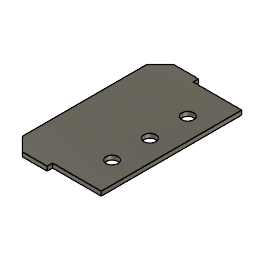
GPL H300 to 300G17_ (Autodesk Fusion 360 design; units mm, degrees)
Autodesk Fusion 360 part; units mm, degrees
sketch "スケッチ1" plane through (0, 0, 0) normal (0, 0, 1) x (1, 0, 0)
  line L0 (-9.5, 140) -> (-80.5, 140)
  line L1 (-80.5, 140) -> (-80.5, -140)
  line L2 (-80.5, -140) -> (-9.5, -140)
  line L3 (80.5, -130) -> (80.5, 130)
  line L4 (74.75, 130) -> (-80.5, -140) construction
  line L5 (-80.5, 140) -> (74.75, -130) construction
  line L6 (-9.5, 140) -> (-9.5, 130)
  line L7 (-9.5, 130) -> (80.5, 130)
  line L8 (-9.5, -140) -> (-9.5, -130)
  line L9 (-9.5, -130) -> (80.5, -130)
  dimension "d2" = 280
  constraint horizontal L0
  constraint perpendicular L0 L1
  constraint parallel L0 L2
  constraint parallel L1 L3
  constraint coincident L4 origin
  constraint coincident L5 origin
  constraint vertical L6
  constraint horizontal L7
  constraint vertical L8
  constraint horizontal L9
  constraint coincident L7 L4.start
  constraint coincident L9 L5.end
  measures "d2" distance of L0.end L1.end
extrude "押し出し1" add sketch "スケッチ1" along normal blind 8
chamfer "面取り1" distance 25 angle 45 2 edges at (-80.5, -140, 4) (-80.5, 140, 4)
sketch "スケッチ2" plane through (0, 0, 8) normal (0, 0, 1) x (-1, 0, 0)
  line L0 (55.5, -140) -> (80.5, -115)
  line L1 (80.5, -115) -> (80.5, 115)
  line L2 (80.5, 115) -> (55.5, 140)
  line L3 (55.5, 140) -> (9.5, 140)
  line L4 (9.5, 140) -> (9.5, 130)
  line L5 (9.5, 130) -> (-80.5, 130)
  line L6 (-80.5, 130) -> (-80.5, -130)
  line L7 (-80.5, -130) -> (9.5, -130)
  line L8 (9.5, -130) -> (9.5, -140)
  line L9 (9.5, -140) -> (55.5, -140)
  line L10 (-80.5, -130) -> (-40.5, -130) construction
  line L11 (-40.5, -130) -> (-40.5, -70) construction
  line L12 (-40.5, -70) -> (-80.5, -70) construction
  line L13 (-80.5, -70) -> (-80.5, -130) construction
  line L14 (-40.5, -70) -> (-40.5, 0) construction
  line L15 (-40.5, 0) -> (-40.5, 70) construction
  point P0 (-40.5, -70)
  point P1 (-40.5, 0)
  point P2 (-40.5, 70)
  dimension "d10" = 40
  dimension "d11" = 60
  dimension "d12" = 70
  dimension "d13" = 70
  constraint horizontal L10
  constraint vertical L11
  constraint horizontal L12
  constraint vertical L13
  constraint coincident L6.end L7.start
  constraint perpendicular L5 L14
  constraint parallel L1 L15
  constraint coincident P0 L11.end
  constraint coincident P1 L14.end
  constraint coincident P2 L15.end
  measures "d10" distance of L6.end L10.end
  measures "d11" distance of L6.end L12.end
  measures "d12" distance of P0 P1
  measures "d13" distance of P1 P2
hole "穴1" at (40.5, 70, 8) at (40.5, 0, 8) at (40.5, -70, 8) direction (0, 0, -1) diameter 22 end through all
